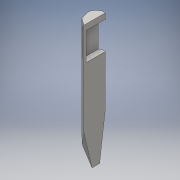
# Autodesk Inventor part: bodyside
Saved by Autodesk Inventor 2016 (Build 200138000, 138)
## iProperties
Created: 2019-01-22
Part Number: bodyside
Material: Generic
Document SubType Name: Modeling
Designer: LinJie
Density: 1 g/cm^3
Appearance: Default
Author: LinJie
Autodesk Inventor part; units mm, degrees
ref_plane "YZ Plane" through (0, 0, 0) normal (1, 0, 0) x (0, 1, 0)
ref_plane "XZ Plane" through (0, 0, 0) normal (0, 1, 0) x (-1, 0, 0)
ref_plane "XY Plane" through (0, 0, 0) normal (0, 0, 1) x (1, 0, 0)
sketch "Sketch1" plane through (0, 0, 0) normal (0, 0, 1) x (1, 0, 0)
  line L0 (-25, -57.5) -> (25, -57.5)
  line L1 (25, -57.5) -> (25, 57.5)
  line L2 (25, 57.5) -> (-25, 57.5)
  line L3 (-25, 57.5) -> (-25, -57.5)
  line L4 (-25, -57.5) -> (25, 57.5) construction
  line L5 (25, -57.5) -> (-25, 57.5) construction
  point P0 (0, 0)
  dimension "d0" = 50
  dimension "d1" = 115
  constraints: 12 end point, 2 midpoint, 2 parallel, 1 horizontal, 1 perpendicular
  measures "d0" distance of L2.end L1.end
  measures "d1" distance of L1.end L0.end
extrude "Extrusion1" add sketch "Sketch1" along normal mid plane 800
sketch "Sketch2" plane through (0, 0, 400) normal (0, 0, 1) x (1, 0, 0)
  line L0 (-25, -57.5) -> (25, -57.5) projected
  line L1 (25, -57.5) -> (25, 57.5) construction
  line L2 (25, 57.5) -> (-25, 57.5) projected
  line L3 (-25, 57.5) -> (-25, -57.5) projected
  line L4 (25, -57.5) -> (86.0387, -57.5) construction
  line L5 (-25, -57.5) -> (25, -57.5) projected
  line L6 (25, -57.5) -> (-11.8618, -31.6891)
  line L7 (25, -57.5) -> (70, -57.5) construction
  line L8 (-11.8618, -31.6891) -> (-22.6774, 1.5979)
  line L9 (-11.8618, -31.6891) -> (23.1382, -31.6891) construction
  arc A0 (-3.649, 50.0435) -> (-22.6774, 1.5979) centre (15.1106, 14.7153) ccw
  line L10 (-3.649, 50.0435) -> (7, 57.5)
  line L11 (-3.649, 50.0435) -> (9.351, 50.0435) construction
  line L12 (25, 57.5) -> (-25, 57.5) projected
  point P0 (0, 0)
  dimension "d5" = 45
  dimension "d6" = 145
  dimension "d7" = 35
  dimension "d8" = 108
  dimension "d9" = 40
  dimension "d10" = 13
  dimension "d11" = 35
  dimension "d12" = 18
  constraints: 14 end point, 4 horizontal, 3 equal length, 2 point on circle, 1 centre point, 1 point on line
  measures "d5" distance of L0.end L6.end
  measures "d6" angle of L7 L6
  measures "d7" distance of L6.end L8.end
  measures "d8" angle of L9 L8
  measures "d9" radius of A0
  measures "d10" distance of L10.start L10.end
  measures "d11" angle of L11 L10
  measures "d12" distance of L1.end L10.end
extrude "Extrusion2" cut sketch "Sketch2" against normal through all
sketch "Sketch3" plane through (0, 0, 0) normal (1, 0, 0) x (0, 1, 0)
  line L0 (57.5, -400) -> (57.5, 400) projected
  line L1 (-57.5, 400) -> (57.5, 400) projected
  line L2 (-57.5, -400) -> (-57.5, 400) projected
  line L3 (57.5, -400) -> (-57.5, -400) projected
  line L4 (-57.5, -400) -> (-57.5, 400) projected
  line L5 (-57.5, -100) -> (12.5, -400)
  line L6 (57.5, -400) -> (-57.5, -400) projected
  point P0 (0, 0)
  dimension "d15" = 300
  dimension "d16" = 70
  constraints: 2 end point, 2 point on line
  measures "d15" distance of L2.start L5.start
  measures "d16" distance from line of L2 L5.end
extrude "Extrusion3" cut sketch "Sketch3" along normal through all both and the other way through all contours L3 L2 L5
sketch "Sketch4" plane through (25, 57.5, 400) normal (1, 0, 0) x (0, 0, -1)
  line L0 (500, -115) -> (800, -45) projected
  line L1 (800, 0) -> (800, -45) projected
  line L2 (800, 0) -> (0, 0) projected
  line L3 (0, -115) -> (0, 0) projected
  line L4 (500, -115) -> (0, -115) projected
  line L5 (800, -45) -> (450, 0)
  point P0 (400, -57.5)
  dimension "d19" = 350
  constraints: 2 end point, 1 point on line
  measures "d19" horizontal distance of L0.end L5.end
extrude "Extrusion4" cut sketch "Sketch4" along normal through all both and the other way through all contours L5 L2 L1
sketch "Sketch5" plane through (0, 0, 0) normal (0, 1, 0) x (-1, 0, 0)
  line L0 (-25, -100) -> (-25, -400) projected
  line L1 (24.8894, -382.7696) -> (24.8894, 400) projected
  line L2 (-25, -400) -> (24.8894, -400)
  line L3 (24.8894, -400) -> (24.8894, 400)
  line L4 (-25, 400) -> (-25, -400)
  line L5 (-7, 400) -> (3.649, 400) projected
  line L6 (24.8894, -100) -> (-55, -400)
  line L7 (-55, -400) -> (-25, -400)
  point P0 (0, 0)
  point P1 (-0.0553, 400)
  dimension "d22" = 30
  dimension "d23" = 300
  constraints: 10 end point, 3 point on line, 2 horizontal, 1 horizontal alignment, 1 parallel, 1 perpendicular
  measures "d22" distance of L0.end L6.end
  measures "d23" distance from line of L2 L6.start
extrude "Extrusion5" cut sketch "Sketch5" along normal through all both and the other way through all
sketch "Sketch6" plane through (7, 57.5, 400) normal (0, 1, 0) x (1, 0, 0)
  line L0 (18, 500) -> (18, 0) projected
  line L1 (18, 30) -> (-12, 30)
  line L2 (-12, 30) -> (-12, 180)
  line L3 (-12, 180) -> (18, 180)
  line L4 (18, 180) -> (18, 30)
  line L5 (18, 0) -> (0, 0) projected
  point P0 (-7, 400)
  dimension "d26" = 30
  dimension "d27" = 150
  dimension "d28" = 30
  constraints: 8 end point, 2 parallel, 1 horizontal, 1 perpendicular, 1 point on line
  measures "d26" distance of L2.end L3.end
  measures "d27" distance between parallel lines of L1 L3
  measures "d28" distance between parallel lines of L5 L1
extrude "Extrusion6" cut sketch "Sketch6" against normal through all
sketch "Sketch7" plane through (-11.8618, -31.6891, -148.9211) normal (-0.5735764, -0.819152, 0) x (0.819152, -0.5735764, 0)
  line L0 (-40.8281, 518.9211) -> (8.3768, 518.9211) projected
  line L1 (-20.9613, 368.9211) -> (45, 368.9211) projected
  line L2 (8.3768, 518.9211) -> (45, 518.9211)
  line L3 (45, 518.9211) -> (45, 368.9211)
  line L4 (45, 368.9211) -> (8.3768, 368.9211)
  line L5 (8.3768, 368.9211) -> (8.3768, 518.9211)
  point P0 (-8.4594, 148.9211)
  constraints: 8 end point, 2 parallel, 1 horizontal, 1 perpendicular
extrude "Extrusion7" add sketch "Sketch7" against normal blind 10
fillet "Fillet1" radius 8 1 edges at (0.7358, -28.3023, 295)
sketch "Sketch8" plane through (25, -57.5, 370) normal (0, 0, 1) x (1, 0, 0)
  line L0 (0, 0) -> (0, 12.2077) projected
  line L1 (0, 0) -> (5.7358, 8.1915) projected
  line L2 (0, 12.2077) -> (5.7358, 8.1915) projected
  point P0 (-25, 57.5)
extrude "Extrusion8" cut sketch "Sketch8" against normal through all
body "Solid1"
